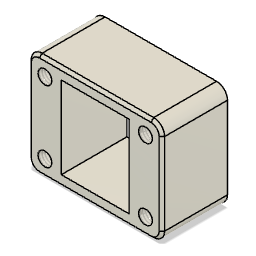
soporte_puentes_H v8 (Autodesk Fusion 360 design; units mm, degrees)
Autodesk Fusion 360 part; units mm, degrees
sketch "Sketch1" plane through (0, 0, 0) normal (0, 0, 1) x (1, 0, 0)
  line L0 (12.2, 9.5) -> (-12.2, 9.5)
  line L1 (-12.2, 9.5) -> (-12.2, -9.5)
  line L2 (-12.2, -9.5) -> (12.2, -9.5)
  line L3 (12.2, -9.5) -> (12.2, 9.5)
  line L4 (12.2, 9.5) -> (-12.2, -9.5) construction
  line L5 (-12.2, 9.5) -> (12.2, -9.5) construction
  line L6 (9.2, 6.5) -> (-9.2, 6.5) construction
  line L7 (-9.2, 6.5) -> (-9.2, -6.5) construction
  line L8 (-9.2, -6.5) -> (9.2, -6.5) construction
  line L9 (9.2, -6.5) -> (9.2, 6.5) construction
  line L10 (9.2, 6.5) -> (-9.2, -6.5) construction
  line L11 (-9.2, 6.5) -> (9.2, -6.5) construction
  circle A0 centre (9.2, 6.5) radius 1.5
  circle A1 centre (-9.2, -6.5) radius 1.5
  line L12 (0, 0) -> (9.2, 0) construction
  circle A2 centre (-9.2, 6.5) radius 1.5
  circle A3 centre (9.2, -6.5) radius 1.5
  line L13 (6.2, 7.5) -> (-6.2, 7.5)
  line L14 (-6.2, 7.5) -> (-6.2, -7.5)
  line L15 (-6.2, -7.5) -> (6.2, -7.5)
  line L16 (6.2, -7.5) -> (6.2, 7.5)
  line L17 (6.2, 7.5) -> (-6.2, -7.5) construction
  line L18 (-6.2, 7.5) -> (6.2, -7.5) construction
  line L19 (0, 0) -> (5.0501, 0) construction
  line L20 (19.3001, 18.69) -> (-9.2, 18.69) construction
  line L21 (-9.2, 18.69) -> (-9.2, -18.69) construction
  line L22 (-9.2, -18.69) -> (19.3001, -18.69) construction
  line L23 (19.3001, -18.69) -> (19.3001, 18.69) construction
  line L24 (19.3001, 18.69) -> (-9.2, -18.69) construction
  line L25 (-9.2, 18.69) -> (19.3001, -18.69) construction
  circle A4 centre (-9.2, 18.69) radius 1.5
  circle A5 centre (-9.2, -18.69) radius 1.5
  line L26 (-12.2, 21.69) -> (-4.2, 21.69)
  line L27 (-4.2, 21.69) -> (-4.2, -21.69)
  line L28 (-4.2, -21.69) -> (-12.2, -21.69)
  line L29 (-12.2, -21.69) -> (-12.2, 21.69)
  point P0 (5.0501, 0)
  dimension "d1" = 18.4
  dimension "d2" = 13
  dimension "d3" = 3
  dimension "d6" = 3
  dimension "d7" = 3
  dimension "d10" = 3
  dimension "d11" = 2
  dimension "d14" = 37.38
  dimension "d15" = 3
  dimension "d16" = 3
  dimension "d17" = 5
  dimension "d18" = 3
  dimension "d19" = 3
  constraint horizontal L0
  constraint perpendicular L0 L1
  constraint parallel L0 L2
  constraint parallel L1 L3
  constraint coincident L4 L12.start
  constraint coincident L5 L12.start
  constraint coincident L12.start L19.start
  constraint horizontal L6
  constraint perpendicular L6 L7
  constraint parallel L6 L8
  constraint parallel L7 L9
  constraint coincident L10 L12.start
  constraint coincident L11 L12.start
  constraint coincident L6.start L9.end
  constraint coincident L7.end L8.start
  constraint midpoint L9 L12.end
  constraint coincident L6.end L7.start
  constraint coincident L8.end L9.start
  constraint equal A0 A2
  constraint equal A0 A1
  constraint equal A0 A3
  constraint horizontal L13
  constraint perpendicular L13 L14
  constraint parallel L13 L15
  constraint parallel L14 L16
  constraint coincident L17 L12.start
  constraint coincident L18 L12.start
  constraint perpendicular L16 L19
  constraint horizontal L20
  constraint perpendicular L20 L21
  constraint parallel L20 L22
  constraint parallel L21 L23
  constraint coincident L24 P0
  constraint coincident L25 P0
  constraint coincident P0 L19.end
  constraint collinear L7 L21
  constraint coincident L20.end L21.start
  constraint coincident L21.end L22.start
  constraint horizontal L26
  constraint vertical L27
  constraint horizontal L28
  constraint vertical L29
  constraint collinear L1 L29
  measures "d1" distance of L6.start L6.end
  measures "d2" distance of L6.start L8.end
  measures "d3" diameter of A0
  measures "d6" distance of L3 L8.end
  measures "d7" distance of L2 L8.end
  measures "d10" distance of L6.start L16
  measures "d11" distance of L0 L13
  measures "d14" distance of L20.end L21.end
  measures "d15" diameter of A4
  measures "d16" diameter of A5
  measures "d17" distance of L21.end L27
  measures "d18" distance of L20.end L26
  measures "d19" distance of L21.end L28
extrude "Extrude1" add sketch "Sketch1" along normal blind 12 contours L0 L2 L3 L13 L15 L16 L27 | L0 L1 L2 L13 L14 L15 L27 L29
fillet "Fillet1" radius 2 4 edges at (12.2, -9.5, 6) (12.2, 9.5, 6) (-12.2, 9.5, 6) (-12.2, -9.5, 6)
thread "Thread1" "ISO Metric profile 3.0 M3x0.5 6H" major diameter 3.086 minor diameter 2.529 pitch 0.5 angle 60 resizes the face on face at (-7.7019, -6.5748, 8) on face at (10.6981, -6.5748, 8) on face at (10.6981, 6.4252, 8) on face at (-7.7019, 6.4252, 8)
sketch "Sketch2" plane through (0, 0, 12) normal (0, 0, 1) x (1, 0, 0)
  line L0 (-12.2, 7.5) -> (-12.2, -7.5)
  line L1 (-10.2, -9.5) -> (10.2, -9.5)
  arc A0 (10.2, -9.5) -> (12.2, -7.5) centre (10.2, -7.5) ccw
  line L2 (12.2, -7.5) -> (12.2, 7.5)
  arc A1 (12.2, 7.5) -> (10.2, 9.5) centre (10.2, 7.5) ccw
  line L3 (10.2, 9.5) -> (-10.2, 9.5)
  line L4 (6.2, 7.5) -> (6.2, -7.5)
  line L5 (6.2, -7.5) -> (-6.2, -7.5)
  line L6 (-6.2, -7.5) -> (-6.2, 7.5)
  line L7 (-6.2, 7.5) -> (6.2, 7.5)
  circle A2 centre (9.2, 6.5) radius 1.2645
  circle A3 centre (-9.2, -6.5) radius 1.2645
  circle A4 centre (9.2, -6.5) radius 1.2645
  circle A5 centre (-9.2, 6.5) radius 1.2645
  line L8 (-12.2, -9.5) -> (-4.2, -9.5)
  line L9 (-4.2, -9.5) -> (-4.2, -14.69)
  line L10 (-4.2, -14.69) -> (-12.2, -14.69)
  line L11 (-12.2, -14.69) -> (-12.2, -9.5)
  line L12 (-4.2, -9.5) -> (-10.2, -9.5)
  line L13 (-4.2, -14.69) -> (-12.2, -14.69)
  line L14 (-12.2, -14.69) -> (-12.2, -11.69)
  line L15 (-12.2, -11.69) -> (-4.2, -11.69)
  line L16 (-4.2, -11.69) -> (-4.2, -14.69)
  line L17 (0, 0) -> (12.2, 0)
  line L18 (-12.2, 14.69) -> (-12.2, 9.5)
  line L19 (-12.2, 9.5) -> (-4.2, 9.5)
  line L20 (-4.2, 14.69) -> (-12.2, 14.69)
  line L21 (-12.2, 14.69) -> (-12.2, 11.69)
  line L22 (-4.2, 11.69) -> (-4.2, 14.69)
  line L23 (-12.2, 11.69) -> (-4.2, 11.69)
  line L24 (-4.2, 9.5) -> (-4.2, 14.69)
  line L25 (-4.2, 9.5) -> (-10.2, 9.5)
  arc A6 (-12.2, -7.5) -> (-10.2, -9.5) centre (-10.2, -7.5) ccw
  arc A7 (-10.2, 9.5) -> (-12.2, 7.5) centre (-10.2, 7.5) ccw
  dimension "d23" = 3
  constraint horizontal L8
  constraint vertical L9
  constraint horizontal L10
  constraint vertical L11
  constraint coincident L0 L8.start
  constraint coincident L1.start L12.end
  constraint horizontal L12
  constraint horizontal L13
  constraint vertical L14
  constraint horizontal L15
  constraint vertical L16
  constraint coincident L11 L14.end
  constraint coincident L17.start origin
  constraint midpoint L2 L17.end
  constraint symmetric L8.start L17 L18.end
  constraint symmetric L8.end L17 L19.end
  constraint symmetric L9.end L17 L20.start
  constraint symmetric L10.end L17 L18.start
  constraint symmetric L1.start L17 L3.end
  constraint symmetric L14.end L17 L21.end
  constraint symmetric L15.end L17 L22.start
  measures "d23" distance of L10 L15
chamfer "Chamfer1" distance 0.5 angle 45 8 edges at (12.2, 0, 12) (11.6142, 8.9142, 12) (0, 9.5, 12) (-11.6142, 8.9142, 12) (-12.2, 0, 12) (-11.6142, -8.9142, 12) (0, -9.5, 12) (11.6142, -8.9142, 12)
equation "d19 = d18"
